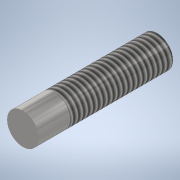
# Autodesk Inventor part: M8_34mmRod
Saved by Autodesk Inventor 2022 (Build 260153000, 153)
## iProperties
Created: 2020-03-30
Part Number: M8_34mmRod
Material: Stainless Steel, Austenitic
Document SubType Name: Modeling
Designer: elmar
Density: 8 g/cm^3
Appearance: Semi-Polished
Author: elmar
Autodesk Inventor part; units mm, degrees
ref_plane "YZ Plane" through (0, 0, 0) normal (1, 0, 0) x (0, 1, 0)
ref_plane "XZ Plane" through (0, 0, 0) normal (0, 1, 0) x (-1, 0, 0)
ref_plane "XY Plane" through (0, 0, 0) normal (0, 0, 1) x (1, 0, 0)
sketch "Sketch1" plane through (0, 0, 0) normal (0, 0, 1) x (1, 0, 0)
  circle A0 centre (0, 0) radius 4
  dimension "d0" = 8
  constraints: 1 centre point, 1 coincident
  measures "d0" diameter of A0
extrude "Extrusion1" add sketch "Sketch1" along normal blind 34
thread "Thread1" size "M8x1.25" class "6g" standard "ANSI Metric M Profile" length 26
equation "\"d12\" = 55deg"
equation "\"Sketch2_Pitch\" = 1.25"
equation "\"d31\" = 55deg"
equation "\"Sketch5_Pitch\" = 1.25"
equation "\"d50\" = 55deg"
equation "\"Sketch8_Pitch\" = 1.25"
equation "\"d69\" = 55deg"
equation "\"Sketch11_Pitch\" = 1.25"
equation "\"d88\" = 55deg"
equation "\"Sketch14_Pitch\" = 1.25"
body "Solid1"
